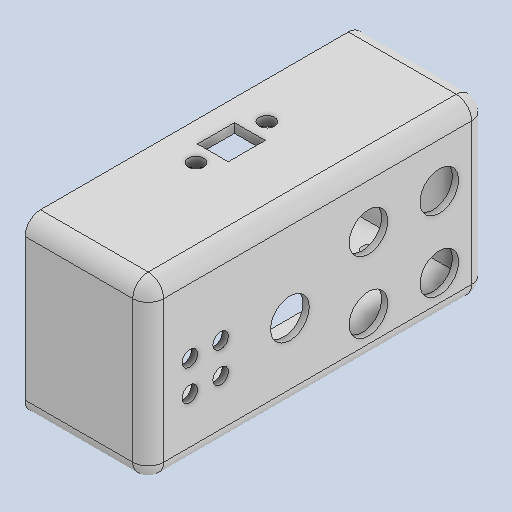
# Autodesk Inventor part: electro_hold
Saved by Autodesk Inventor 2025 (Build 290162000, 162)
## iProperties
Created: 2025-08-20
Part Number: electro_hold
Material: Generic
Document SubType Name: Modeling
Designer: Pravoslav
Density: 1 g/cm^3
Appearance: Default
Author: Pravoslav
Autodesk Inventor part; units mm, degrees
ref_plane "YZ Plane" through (0, 0, 0) normal (1, 0, 0) x (0, 1, 0)
ref_plane "XZ Plane" through (0, 0, 0) normal (0, 1, 0) x (-1, 0, 0)
ref_plane "XY Plane" through (0, 0, 0) normal (0, 0, 1) x (1, 0, 0)
sketch "Sketch1" plane through (0, 0, 0) normal (0, 1, 0) x (-1, 0, 0)
  circle A0 centre (0, 45) radius 2.5
  circle A1 centre (0, -45) radius 2.5
  line L0 (12, 55) -> (-28, 55)
  line L1 (-28, 55) -> (-28, -55)
  line L2 (-28, -55) -> (12, -55)
  line L3 (12, -55) -> (12, 55)
  line L4 (-6, -35) -> (6, -35)
  line L5 (6, -35) -> (6, 35)
  line L6 (6, 35) -> (-6, 35)
  line L7 (-6, 35) -> (-6, -35)
  point P0 (0, 0)
  point P1 (0, -35)
  point P2 (0, 35)
  dimension "d0" = 5
  dimension "d1" = 5
  dimension "d2" = 90
  dimension "d3" = 45
  dimension "d4" = 40
  dimension "d6" = 110
  dimension "d7" = 55
  dimension "d36" = 70
  dimension "d37" = 12
  dimension "d38" = 35
  dimension "d39" = 0
  dimension "d40" = 28
  dimension "d42" = 0
  dimension "d52" = 0
  constraints: 16 end point, 4 parallel, 2 centre point, 2 horizontal, 2 midpoint, 2 perpendicular
  measures "d0" diameter of A0
  measures "d1" diameter of A1
  measures "d2" distance of A1.centre A0.centre
  measures "d3" distance of point (0, 0) A1.centre
  measures "d4" distance between parallel lines of L1 L3
  measures "d6" distance between parallel lines of L2 L0
  measures "d7" distance from line of point (0, 0) L0
  measures "d36" distance between parallel lines of L6 L4
  measures "d37" distance between parallel lines of L5 L7
  measures "d38" distance from line of point (0, 0) L4
  measures "d39" horizontal distance of A1.centre point (0, -35)
  measures "d40" distance from line of L1 A1.centre
  measures "d42" horizontal distance of A1.centre point (0, 0)
  measures "d52" horizontal distance of point (0, 35) A0.centre
extrude "Extrusion1" add sketch "Sketch1" along normal blind 3
sketch "Sketch2" plane through (0, 3, 0) normal (0, 1, 0) x (1, 0, 0)
  line L0 (-12, -55) -> (28, -55) projected
  line L1 (-12, 55) -> (-12, -55) projected
  line L2 (28, -55) -> (-12, -55)
  line L3 (-12, -55) -> (-12, -53)
  line L4 (-12, -53) -> (28, -53)
  line L5 (28, -53) -> (28, -55)
  line L6 (28, 55) -> (-12, 55) projected
  line L7 (28, -55) -> (26, -55)
  line L8 (26, -55) -> (26, 55)
  line L9 (26, 55) -> (28, 55)
  line L10 (28, 55) -> (28, -55)
  line L11 (28, 55) -> (-12, 55)
  line L12 (-12, 55) -> (-12, 53)
  line L13 (-12, 53) -> (28, 53)
  line L14 (28, 53) -> (28, 55)
  point P0 (0, 0)
  point P1 (-12, 53)
  point P2 (26, 53)
  point P3 (26, -53)
  dimension "d10" = 2
  dimension "d11" = 2
  dimension "d12" = 2
  constraints: 24 end point, 6 parallel, 3 horizontal, 3 perpendicular, 3 point on line
  measures "d10" distance of L2.end L3.end
  measures "d11" distance of L8.end L9.end
  measures "d12" distance of L12.end L11.end
extrude "Extrusion2" add sketch "Sketch2" along normal blind 50 contours L1 L4 L8 L0 | L8 L4 L5 L0 | L8 L13 L10 L4 | L1 L6 L8 L13 | L8 L6 L10 L13
sketch "Sketch3" plane through (28, 0, 55) normal (1, 0, 0) x (0, 0, -1)
  line L0 (94.5, 13.5) -> (71.5, 13.5)
  line L1 (71.5, 13.5) -> (71.5, 36.5)
  line L2 (71.5, 36.5) -> (94.5, 36.5)
  line L3 (94.5, 36.5) -> (94.5, 13.5)
  line L4 (94.5, 13.5) -> (71.5, 36.5) construction
  line L5 (71.5, 13.5) -> (94.5, 36.5) construction
  circle A0 centre (94.5, 13.5) radius 6.25
  circle A1 centre (71.5, 13.5) radius 6.25
  circle A2 centre (94.5, 36.5) radius 6.25
  circle A3 centre (71.5, 36.5) radius 6.25
  line L6 (23.5, 20) -> (13.5, 20)
  line L7 (13.5, 20) -> (13.5, 30)
  line L8 (13.5, 30) -> (23.5, 30)
  line L9 (23.5, 30) -> (23.5, 20)
  line L10 (23.5, 20) -> (13.5, 30) construction
  line L11 (13.5, 20) -> (23.5, 30) construction
  circle A4 centre (23.5, 20) radius 2.5
  circle A5 centre (13.5, 20) radius 2.5
  circle A6 centre (13.5, 30) radius 2.5
  circle A7 centre (23.5, 30) radius 2.5
  circle A8 centre (46, 25) radius 6.25
  line L12 (0, 0) -> (110, 0) projected
  line L13 (110, 0) -> (110, 53) projected
  point P0 (55, 0)
  point P1 (83, 25)
  point P2 (18.5, 25)
  dimension "d15" = 23
  dimension "d16" = 23
  dimension "d17" = 12.5
  dimension "d18" = 12.5
  dimension "d19" = 12.5
  dimension "d20" = 12.5
  dimension "d21" = 10
  dimension "d22" = 10
  dimension "d23" = 5
  dimension "d24" = 5
  dimension "d25" = 5
  dimension "d26" = 5
  dimension "d27" = 12.5
  dimension "d28" = 25
  dimension "d29" = 25
  dimension "d30" = 25
  dimension "d31" = 27
  dimension "d32" = 37
  dimension "d33" = 27.5
  constraints: 24 end point, 9 centre point, 8 coincident, 4 midpoint, 4 parallel, 2 horizontal, 2 perpendicular
  measures "d15" distance of L1.end L2.end
  measures "d16" distance of L0.end L1.end
  measures "d17" diameter of A0
  measures "d18" diameter of A1
  measures "d19" diameter of A2
  measures "d20" diameter of A3
  measures "d21" distance of L7.end L8.end
  measures "d22" distance of L6.end L7.end
  measures "d23" diameter of A4
  measures "d24" diameter of A5
  measures "d25" diameter of A6
  measures "d26" diameter of A7
  measures "d27" diameter of A8
  measures "d28" distance from line of L12 point (83, 25)
  measures "d29" distance from line of L12 A8.centre
  measures "d30" distance from line of L12 point (18.5, 25)
  measures "d31" distance from line of L13 point (83, 25)
  measures "d32" distance of point (83, 25) A8.centre
  measures "d33" distance of A8.centre point (18.5, 25)
extrude "Extrusion3" cut sketch "Sketch3" against normal through all contours A1 L1 L0 | L0 L1 A1 | A0 L3 L0 | L0 L3 A0 | A3 L2 L1 | L1 L2 A3 | A2 L2 L3 | L3 L2 A2 | A5 L7 L6 | L6 L7 A5 | A4 L9 L6 | L6 L9 A4 | A6 L8 L7 | L7 L8 A6 | A7 L8 L9 | L9 L8 A7 | A8
sketch "Sketch4" plane through (0, 53, 0) normal (0, 1, 0) x (1, 0, 0)
  line L0 (28, 55) -> (-12, 55) projected
  line L1 (28, 55) -> (-12, 55)
  line L2 (-12, 55) -> (-12, -55)
  line L3 (-12, -55) -> (28, -55)
  line L4 (28, -55) -> (28, 55)
  line L5 (5, 6) -> (-5, 6)
  line L6 (-5, 6) -> (-5, -6)
  line L7 (-5, -6) -> (5, -6)
  line L8 (5, -6) -> (5, 6)
  line L9 (5, 6) -> (-5, -6) construction
  line L10 (-5, 6) -> (5, -6) construction
  circle A0 centre (0, 11.5) radius 2.5
  circle A1 centre (0, -11.5) radius 2.5
  point P0 (0, 0)
  dimension "d43" = 10
  dimension "d44" = 12
  dimension "d45" = 5
  dimension "d46" = 5
  dimension "d47" = 23
  dimension "d48" = 11.5
  constraints: 20 end point, 4 parallel, 2 centre point, 2 horizontal, 2 midpoint, 2 perpendicular
  measures "d43" distance of L7.end L6.end
  measures "d44" distance of L6.end L5.end
  measures "d45" diameter of A0
  measures "d46" diameter of A1
  measures "d47" distance of A1.centre A0.centre
  measures "d48" distance of point (0, 0) A0.centre
extrude "Extrusion4" add sketch "Sketch4" along normal blind 3
fillet "Fillet1" radius 5 8 edges at (28, 0, 0) (28, 28, -55) (8, 0, -55) (8, 0, 55) (28, 28, 55) (28, 56, 0) (8, 56, -55) (8, 56, 55)
sketch "Sketch5" plane through (-12, 0, -50) normal (-1, 0, 0) x (0, 0, 1)
  line L0 (-3, 53) -> (103, 53) projected
  line L1 (103, 53) -> (85.5, 53)
  line L2 (85.5, 53) -> (85.5, 35.5)
  line L3 (85.5, 35.5) -> (103, 35.5)
  line L4 (103, 35.5) -> (103, 53)
  line L5 (-3, 53) -> (14.5, 53)
  line L6 (14.5, 53) -> (14.5, 35.5)
  line L7 (14.5, 35.5) -> (-3, 35.5)
  line L8 (-3, 35.5) -> (-3, 53)
  circle A0 centre (94.25, 44.25) radius 2.5
  circle A1 centre (5.75, 44.25) radius 2.5
  point P0 (50, 0)
  point P1 (14.5, 53)
  dimension "d54" = 17.5
  dimension "d55" = 17.5
  dimension "d56" = 17.5
  dimension "d57" = 17.5
  dimension "d58" = 5
  dimension "d59" = 5
  dimension "d60" = 8.75
  dimension "d61" = 8.75
  dimension "d62" = 8.75
  dimension "d63" = 8.75
  constraints: 16 end point, 4 parallel, 2 centre point, 2 horizontal, 2 perpendicular
  measures "d54" distance of L3.end L2.end
  measures "d55" distance of L2.end L1.end
  measures "d56" distance of L6.end L7.end
  measures "d57" distance of L5.end L6.end
  measures "d58" diameter of A0
  measures "d59" diameter of A1
  measures "d60" distance from line of L7 A1.centre
  measures "d61" distance from line of L6 A1.centre
  measures "d62" distance from line of L3 A0.centre
  measures "d63" distance from line of L4 A0.centre
extrude "Extrusion5" add sketch "Sketch5" against normal blind 3
fillet "Fillet2" radius 5 6 edges at (-10.5, 35.5, 53) (-10.5, 35.5, 35.5) (-10.5, 53, 35.5) (-10.5, 53, -35.5) (-10.5, 35.5, -35.5) (-10.5, 35.5, -53)
body "Solid1"
